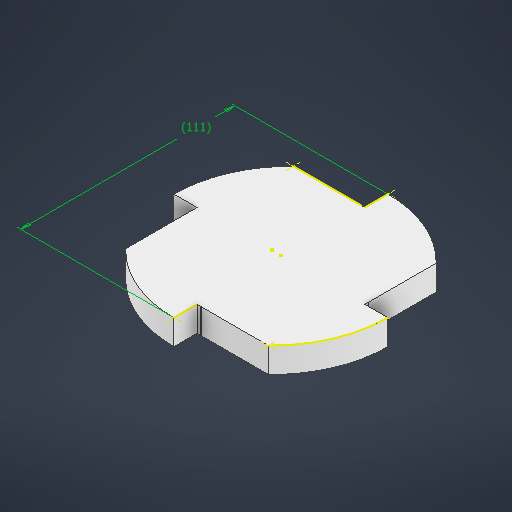
# Autodesk Inventor part: Carbon_Fibre
Saved by Autodesk Inventor 2026.2 (Build 302298000, 298)
## iProperties
Created: 2025-12-09
Part Number: Carbon_Fibre
Material: PC/ABS Plastic
Document SubType Name: Modeling
Designer: Thoma
Density: 1.1 g/cm^3
Appearance: Smooth - White
Author: Thoma
Autodesk Inventor part; units mm, degrees
ref_plane "YZ Plane" through (0, 0, 0) normal (1, 0, 0) x (0, 1, 0)
ref_plane "XZ Plane" through (0, 0, 0) normal (0, 1, 0) x (-1, 0, 0)
ref_plane "XY Plane" through (0, 0, 0) normal (0, 0, 1) x (1, 0, 0)
sketch "Sketch1" plane through (0, 0, 0) normal (0, 1, 0) x (-1, 0, 0)
  circle A0 centre (0, 0) radius 43.5
  dimension "d0" = 87
  constraints: 1 centre point, 1 coincident
  measures "d0" diameter of A0
extrude "Extrusion1" add sketch "Sketch1" along normal blind 13
sketch "Sketch2" plane through (0, 13, 0) normal (0, 1, 0) x (1, 0, 0)
  circle A0 centre (0, 0) radius 43.5 projected
  line L0 (0, 43.5) -> (0, 55.5)
  line L1 (-43.5, 0) -> (-55.5, 0)
  line L2 (0, -43.5) -> (0, -55.5)
  line L3 (43.5, 0) -> (55.5, 0)
  line L4 (43.454, 2) -> (55.5, 2)
  line L5 (55.5, 0) -> (55.5, 2)
  circle A1 centre (0, 0) radius 43.5 projected
  line L6 (43.5, 0) -> (43.5, 37)
  arc A2 (43.5, 37) -> (0, 55.5) centre (0, -4.8919) ccw
  line L7 (-43.5, 0) -> (-55.5, 0)
  arc A3 (-37, 43.5) -> (-55.5, 0) centre (4.8919, 0) ccw
  line L8 (0, 43.5) -> (-37, 43.5)
  line L9 (-2, 43.454) -> (-2, 55.5)
  line L10 (0, 43.5) -> (0, 55.5)
  line L11 (0, 55.5) -> (-2, 55.5)
  line L12 (0, -43.5) -> (0, -55.5)
  arc A4 (-43.5, -37) -> (0, -55.5) centre (0, 4.8919) ccw
  line L13 (-43.5, 0) -> (-43.5, -37)
  line L14 (-43.454, -2) -> (-55.5, -2)
  line L15 (-43.5, 0) -> (-55.5, 0)
  line L16 (-55.5, 0) -> (-55.5, -2)
  line L17 (43.5, 0) -> (55.5, 0)
  arc A5 (37, -43.5) -> (55.5, 0) centre (-4.8919, 0) ccw
  line L18 (0, -43.5) -> (37, -43.5)
  line L19 (2, -43.454) -> (2, -55.5)
  line L20 (0, -43.5) -> (0, -55.5)
  line L21 (0, -55.5) -> (2, -55.5)
  point P0 (0, -55.5)
  point P1 (-43.5, -2)
  point P2 (-55.5, 0)
  point P3 (-2, 43.5)
  point P4 (55.5, 0)
  point P5 (43.5, 0)
  point P6 (2, -43.5)
  point P7 (43.5, 2)
  dimension "d3" = 12
  dimension "d6" = 360
  dimension "d8" = 2
  dimension "d10" = 35
  dimension "d13" = 360
  constraints: 44 end point, 10 point on circle, 4 centre point, 2 tangent, 2 vertical, 1 horizontal, 1 perpendicular, 70 other
  measures "d3" distance of L0.start L0.end
  measures "d8" distance between parallel lines of L4 L3
  measures "d10" distance of L6.end L4.start
extrude "Extrusion2" add sketch "Sketch2" against normal blind 13 contours L3 A5 L18 L19 A0 | A0 L0 A2 L6 L4 | L2 A4 L13 L14 A0 | A0 L1 A3 L8 L9
sketch "Sketch3" plane through (0, 13, 0) normal (0, 1, 0) x (1, 0, 0)
  line L0 (0, -43.5) -> (0, -55.5) projected
  line L1 (0, 43.5) -> (0, 55.5) projected
  line L2 (-37, 43.5) -> (-2, 43.5) projected
  arc A0 (37, -43.5) -> (55.5, 0) centre (-4.8919, 0) ccw projected
  point P0 (0, 0)
  dimension "d17" = 111
  measures "d17" distance of L1.end L0.end
body "Solid1"
